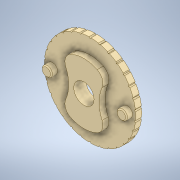
# Autodesk Inventor part: manivela
Saved by Autodesk Inventor 2022 (Build 260153000, 153)
## iProperties
Created: 2023-03-13
Part Number: manivela
Material: Genérico
Document SubType Name: Modeling
Designer: jpjoa
Density: 1 g/cm^3
Appearance: Bege
Author: jpjoa
Autodesk Inventor part; units mm, degrees
ref_plane "YZ Plane" through (0, 0, 0) normal (1, 0, 0) x (0, 1, 0)
ref_plane "XZ Plane" through (0, 0, 0) normal (0, 1, 0) x (-1, 0, 0)
ref_plane "XY Plane" through (0, 0, 0) normal (0, 0, 1) x (1, 0, 0)
sketch "Esboço1" plane through (0, 0, 0) normal (0, 0, 1) x (1, 0, 0)
  circle A0 centre (0, 0) radius 10
  circle A1 centre (0, 0) radius 30
  arc A2 (21.75, 20.6625) -> (21.75, -20.6625) centre (50, 0) ccw
  circle A3 centre (0, 0) radius 45
  arc A4 (-21.75, -20.6625) -> (-21.75, 20.6625) centre (-50, 0) ccw
  circle A5 centre (37, 0) radius 5
  circle A6 centre (-37, 0) radius 5
  dimension "d0" = 20
  dimension "d1" = 60
  dimension "d2" = 70
  dimension "d3" = 90
  dimension "d4" = 50
  dimension "d5" = 70
  dimension "d6" = 50
  dimension "d7" = 10
  dimension "d8" = 10
  dimension "d9" = 74
  dimension "d10" = 37
  constraints: 8 point on circle, 7 centre point, 4 horizontal alignment, 3 coincident
  measures "d0" diameter of A0
  measures "d1" diameter of A1
  measures "d2" diameter of A2
  measures "d3" diameter of A3
  measures "d4" distance of A2.centre point (0, 0)
  measures "d5" diameter of A4
  measures "d6" distance of point (0, 0) A4.centre
  measures "d7" diameter of A5
  measures "d8" diameter of A6
  measures "d9" distance of A5.centre A6.centre
  measures "d10" distance of point (0, 0) A6.centre
extrude "Extrusão1" add sketch "Esboço1" along normal blind 6 contours A1 A2 | A4 A1 | A3
extrude "Extrusão2" add sketch "Esboço1" along normal blind 12 contours A2 A1 A4 | A5 | A6
fillet "Arredondamento1" radius 10 4 edges at (21.75, 20.6625, 9) (21.75, -20.6625, 9) (-21.75, 20.6625, 9) (-21.75, -20.6625, 9)
chamfer "Chanfro1" distance 1 angle 45 2 edges at (-42, 0, 12) (32, 0, 12)
sketch "Esboço2" plane through (0, 0, 6) normal (0, 0, 1) x (1, 0, 0)
  line L0 (1, 45) -> (-1, 45)
  line L1 (-1, 45) -> (0, 44)
  line L2 (0, 44) -> (1, 45)
  circle A0 centre (0, 0) radius 45 projected
  point P0 (0, 45)
  point P1 (-0.9891, 44.9891)
  point P2 (0.9891, 44.9891)
  dimension "d24" = 2
  constraints: 6 end point, 2 vertical alignment, 1 horizontal, 1 midpoint, 1 perpendicular, 1 tangent
  measures "d24" distance of L0.start L0.end
extrude "Extrusão3" cut sketch "Esboço2" against normal through all contours A0 L2 L1 picked at (0.5495, 44.6614)
pattern_circular "Padrão circular1" count 30 over 360 about axis through (0, 0, 0) along (0, 0, 1) of "Extrusão3"
